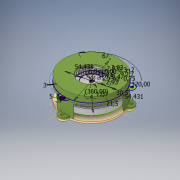
# Autodesk Inventor part: HarmonicDriveProto2
Saved by Autodesk Inventor 2018.3 (Build 223284000, 284)
## iProperties
Created: 2018-06-22
Part Number: HarmonicDriveProto2
Material: Generisch
Document SubType Name: Modeling
Designer: JochenAlt
Density: 1 g/cm^3
Appearance: Vorgabe
Author: JochenAlt
Autodesk Inventor part; units mm, degrees
note: some values were not read from the file. Chosen so that the rebuilt part matches the saved one: sketch regions of "Extrusion4".
(part 1 of 2)
ref_plane "YZ Plane" through (0, 0, 0) normal (1, 0, 0) x (0, 1, 0)
sketch "Riemen" plane through (0, 0, 0) normal (0, 0, 1) x (1, 0, 0)
  circle A0 centre (0, 0) radius 27.4555 construction
  circle A1 centre (0, 0) radius 26.4655
  circle A2 centre (0, 0) radius 29.1655 construction
  line L0 (0, 43.4877) -> (0, -41.2966) construction
  line L1 (-40.8583, 0) -> (40.8583, 0) construction
  line L2 (0, 0) -> (5.5324, 31.3756) construction
  circle A3 centre (0, 0) radius 27.2155 construction
  line L3 (-1.465, 27.176) -> (1.465, 27.176) construction
  line L4 (3.2763, 27.0176) -> (6.1618, 26.5088) construction
  arc A4 (4.2713, 28.7473) -> (3.3977, 27.4807) centre (6.1618, 26.5088) ccw
  arc A5 (0.5608, 29.1601) -> (0, 29.1655) centre (0, 0) ccw
  arc A6 (5.0645, 28.7224) -> (4.5113, 28.8145) centre (0, 0) ccw
  arc A7 (3.081, 27.2821) -> (1.7033, 27.4026) centre (0, 0) ccw
  arc A8 (1.4259, 27.6532) -> (0.7855, 29.0523) centre (-1.465, 27.176) ccw
  arc A9 (0.7855, 29.0523) -> (0.5608, 29.1601) centre (0.5551, 28.8602) ccw
  arc A10 (1.4259, 27.6532) -> (1.7033, 27.4026) centre (1.7219, 27.702) ccw
  arc A11 (3.081, 27.2821) -> (3.3977, 27.4807) centre (3.1147, 27.5802) ccw
  arc A12 (4.5113, 28.8145) -> (4.2713, 28.7473) centre (4.4649, 28.5181) ccw
  line L5 (0, 0) -> (2.7172, 31.0575) construction
  arc A13 (-4.5113, 28.8145) -> (-5.0645, 28.7224) centre (0, 0) ccw
  arc A14 (-4.2713, 28.7473) -> (-4.5113, 28.8145) centre (-4.4649, 28.5181) ccw
  arc A15 (-3.3977, 27.4807) -> (-4.2713, 28.7473) centre (-6.1618, 26.5088) ccw
  arc A16 (-1.7033, 27.4026) -> (-3.081, 27.2821) centre (0, 0) ccw
  arc A17 (-1.7033, 27.4026) -> (-1.4259, 27.6532) centre (-1.7219, 27.702) ccw
  arc A18 (-0.7855, 29.0523) -> (-1.4259, 27.6532) centre (1.465, 27.176) ccw
  arc A19 (-0.5608, 29.1601) -> (-0.7855, 29.0523) centre (-0.5551, 28.8602) ccw
  arc A20 (0, 29.1655) -> (-0.5608, 29.1601) centre (0, 0) ccw
  arc A21 (-3.3977, 27.4807) -> (-3.081, 27.2821) centre (-3.1147, 27.5802) ccw
  arc A22 (-9.4463, 27.5933) -> (-9.9752, 27.4066) centre (0, 0) ccw
  arc A23 (-9.1983, 27.5688) -> (-9.4463, 27.5933) centre (-9.3492, 27.3095) ccw
  arc A24 (-8.118, 26.4732) -> (-9.1983, 27.5688) centre (-10.6714, 25.0361) ccw
  arc A25 (-6.4358, 26.6905) -> (-7.7717, 26.3326) centre (0, 0) ccw
  arc A26 (-6.4358, 26.6905) -> (-6.2061, 26.9855) centre (-6.5061, 26.9822) ccw
  arc A27 (-5.8184, 28.4745) -> (-6.2061, 26.9855) centre (-3.2763, 27.0176) ccw
  arc A28 (-5.6159, 28.6197) -> (-5.8184, 28.4745) centre (-5.5581, 28.3253) ccw
  arc A29 (-5.0645, 28.7224) -> (-5.6159, 28.6197) centre (0, 0) ccw
  arc A30 (-8.118, 26.4732) -> (-7.7717, 26.3326) centre (-7.8566, 26.6203) ccw
  arc A31 (-14.0944, 25.5338) -> (-14.5827, 25.2581) centre (0, 0) ccw
  arc A32 (-13.8459, 25.5527) -> (-14.0944, 25.5338) centre (-13.9494, 25.2712) ccw
  arc A33 (-12.5917, 24.6613) -> (-13.8459, 25.5527) centre (-14.8567, 22.8026) ccw
  arc A34 (-10.9728, 25.1675) -> (-12.2262, 24.583) centre (0, 0) ccw
  arc A35 (-10.9728, 25.1675) -> (-10.7978, 25.4978) centre (-11.0927, 25.4425) ccw
  arc A36 (-10.6746, 27.0315) -> (-10.7978, 25.4978) centre (-7.9181, 26.0382) ccw
  arc A37 (-10.5003, 27.2097) -> (-10.6746, 27.0315) centre (-10.3923, 26.9298) ccw
  arc A38 (-9.9752, 27.4066) -> (-10.5003, 27.2097) centre (0, 0) ccw
  arc A39 (-12.5917, 24.6613) -> (-12.2262, 24.583) centre (-12.3598, 24.8516) ccw
  arc A40 (-18.3141, 22.6984) -> (-18.7472, 22.3421) centre (0, 0) ccw
  arc A41 (-18.0727, 22.7602) -> (-18.3141, 22.6984) centre (-18.1258, 22.4649) ccw
  arc A42 (-16.6828, 22.1001) -> (-18.0727, 22.7602) centre (-18.5907, 19.8764) ccw
  arc A43 (-15.1764, 22.8797) -> (-16.3093, 22.0865) centre (0, 0) ccw
  arc A44 (-15.1764, 22.8797) -> (-15.0614, 23.2354) centre (-15.3422, 23.1297) ccw
  arc A45 (-15.2064, 24.7673) -> (-15.0614, 23.2354) centre (-12.3193, 24.2676) ccw
  arc A46 (-15.0657, 24.973) -> (-15.2064, 24.7673) centre (-14.9108, 24.7161) ccw
  arc A47 (-14.5827, 25.2581) -> (-15.0657, 24.973) centre (0, 0) ccw
  arc A48 (-16.6828, 22.1001) -> (-16.3093, 22.0865) centre (-16.4875, 22.3278) ccw
  arc A49 (-21.9774, 19.1734) -> (-22.3421, 18.7472) centre (0, 0) ccw
  arc A50 (-21.7504, 19.2761) -> (-21.9774, 19.1734) centre (-21.7514, 18.9762) ccw
  arc A51 (-20.267, 18.8674) -> (-21.7504, 19.2761) centre (-21.7597, 16.3462) ccw
  arc A52 (-18.9188, 19.8968) -> (-19.8968, 18.9188) centre (0, 0) ccw
  arc A53 (-18.9188, 19.8968) -> (-18.8674, 20.267) centre (-19.1256, 20.1142) ccw
  arc A54 (-19.2761, 21.7504) -> (-18.8674, 20.267) centre (-16.3462, 21.7597) ccw
  arc A55 (-19.1734, 21.9774) -> (-19.2761, 21.7504) centre (-18.9762, 21.7514) ccw
  arc A56 (-18.7472, 22.3421) -> (-19.1734, 21.9774) centre (0, 0) ccw
  arc A57 (-20.267, 18.8674) -> (-19.8968, 18.9188) centre (-20.1142, 19.1256) ccw
  arc A58 (-24.973, 15.0657) -> (-25.2581, 14.5827) centre (0, 0) ccw
  arc A59 (-24.7673, 15.2064) -> (-24.973, 15.0657) centre (-24.7161, 14.9108) ccw
  arc A60 (-23.2354, 15.0614) -> (-24.7673, 15.2064) centre (-24.2676, 12.3193) ccw
  arc A61 (-22.0865, 16.3093) -> (-22.8797, 15.1764) centre (0, 0) ccw
  arc A62 (-22.0865, 16.3093) -> (-22.1001, 16.6828) centre (-22.3278, 16.4875) ccw
  arc A63 (-22.7602, 18.0727) -> (-22.1001, 16.6828) centre (-19.8764, 18.5907) ccw
  arc A64 (-22.6984, 18.3141) -> (-22.7602, 18.0727) centre (-22.4649, 18.1258) ccw
  arc A65 (-22.3421, 18.7472) -> (-22.6984, 18.3141) centre (0, 0) ccw
  arc A66 (-23.2354, 15.0614) -> (-22.8797, 15.1764) centre (-23.1297, 15.3422) ccw
  arc A67 (-27.2097, 10.5003) -> (-27.4066, 9.9752) centre (0, 0) ccw
  arc A68 (-27.0315, 10.6746) -> (-27.2097, 10.5003) centre (-26.9298, 10.3923) ccw
  arc A69 (-25.4978, 10.7978) -> (-27.0315, 10.6746) centre (-26.0382, 7.9181) ccw
  arc A70 (-24.583, 12.2262) -> (-25.1675, 10.9728) centre (0, 0) ccw
  arc A71 (-24.583, 12.2262) -> (-24.6613, 12.5917) centre (-24.8516, 12.3598) ccw
  arc A72 (-25.5527, 13.8459) -> (-24.6613, 12.5917) centre (-22.8026, 14.8567) ccw
  arc A73 (-25.5338, 14.0944) -> (-25.5527, 13.8459) centre (-25.2712, 13.9494) ccw
  arc A74 (-25.2581, 14.5827) -> (-25.5338, 14.0944) centre (0, 0) ccw
  arc A75 (-25.4978, 10.7978) -> (-25.1675, 10.9728) centre (-25.4425, 11.0927) ccw
  arc A76 (-28.6197, 5.6159) -> (-28.7224, 5.0645) centre (0, 0) ccw
  arc A77 (-28.4745, 5.8184) -> (-28.6197, 5.6159) centre (-28.3253, 5.5581) ccw
  arc A78 (-26.9855, 6.2061) -> (-28.4745, 5.8184) centre (-27.0176, 3.2763) ccw
  arc A79 (-26.3326, 7.7717) -> (-26.6905, 6.4358) centre (0, 0) ccw
  arc A80 (-26.3326, 7.7717) -> (-26.4732, 8.118) centre (-26.6203, 7.8566) ccw
  arc A81 (-27.5688, 9.1983) -> (-26.4732, 8.118) centre (-25.0361, 10.6714) ccw
  arc A82 (-27.5933, 9.4463) -> (-27.5688, 9.1983) centre (-27.3095, 9.3492) ccw
  arc A83 (-27.4066, 9.9752) -> (-27.5933, 9.4463) centre (0, 0) ccw
  arc A84 (-26.9855, 6.2061) -> (-26.6905, 6.4358) centre (-26.9822, 6.5061) ccw
  arc A85 (-29.1601, 0.5608) -> (-29.1655, 0) centre (0, 0) ccw
  arc A86 (-29.0523, 0.7855) -> (-29.1601, 0.5608) centre (-28.8602, 0.5551) ccw
  arc A87 (-27.6532, 1.4259) -> (-29.0523, 0.7855) centre (-27.176, -1.465) ccw
  arc A88 (-27.2821, 3.081) -> (-27.4026, 1.7033) centre (0, 0) ccw
  arc A89 (-27.2821, 3.081) -> (-27.4807, 3.3977) centre (-27.5802, 3.1147) ccw
  arc A90 (-28.7473, 4.2713) -> (-27.4807, 3.3977) centre (-26.5088, 6.1618) ccw
  arc A91 (-28.8145, 4.5113) -> (-28.7473, 4.2713) centre (-28.5181, 4.4649) ccw
  arc A92 (-28.7224, 5.0645) -> (-28.8145, 4.5113) centre (0, 0) ccw
  arc A93 (-27.6532, 1.4259) -> (-27.4026, 1.7033) centre (-27.702, 1.7219) ccw
  arc A94 (-28.8145, -4.5113) -> (-28.7224, -5.0645) centre (0, 0) ccw
  arc A95 (-28.7473, -4.2713) -> (-28.8145, -4.5113) centre (-28.5181, -4.4649) ccw
  arc A96 (-27.4807, -3.3977) -> (-28.7473, -4.2713) centre (-26.5088, -6.1618) ccw
  arc A97 (-27.4026, -1.7033) -> (-27.2821, -3.081) centre (0, 0) ccw
  arc A98 (-27.4026, -1.7033) -> (-27.6532, -1.4259) centre (-27.702, -1.7219) ccw
  arc A99 (-29.0523, -0.7855) -> (-27.6532, -1.4259) centre (-27.176, 1.465) ccw
  arc A100 (-29.1601, -0.5608) -> (-29.0523, -0.7855) centre (-28.8602, -0.5551) ccw
  arc A101 (-29.1655, 0) -> (-29.1601, -0.5608) centre (0, 0) ccw
  arc A102 (-27.4807, -3.3977) -> (-27.2821, -3.081) centre (-27.5802, -3.1147) ccw
  arc A103 (-27.5933, -9.4463) -> (-27.4066, -9.9752) centre (0, 0) ccw
  arc A104 (-27.5688, -9.1983) -> (-27.5933, -9.4463) centre (-27.3095, -9.3492) ccw
  arc A105 (-26.4732, -8.118) -> (-27.5688, -9.1983) centre (-25.0361, -10.6714) ccw
  arc A106 (-26.6905, -6.4358) -> (-26.3326, -7.7717) centre (0, 0) ccw
  arc A107 (-26.6905, -6.4358) -> (-26.9855, -6.2061) centre (-26.9822, -6.5061) ccw
  arc A108 (-28.4745, -5.8184) -> (-26.9855, -6.2061) centre (-27.0176, -3.2763) ccw
  arc A109 (-28.6197, -5.6159) -> (-28.4745, -5.8184) centre (-28.3253, -5.5581) ccw
  arc A110 (-28.7224, -5.0645) -> (-28.6197, -5.6159) centre (0, 0) ccw
  arc A111 (-26.4732, -8.118) -> (-26.3326, -7.7717) centre (-26.6203, -7.8566) ccw
  arc A112 (-25.5338, -14.0944) -> (-25.2581, -14.5827) centre (0, 0) ccw
  arc A113 (-25.5527, -13.8459) -> (-25.5338, -14.0944) centre (-25.2712, -13.9494) ccw
  arc A114 (-24.6613, -12.5917) -> (-25.5527, -13.8459) centre (-22.8026, -14.8567) ccw
  arc A115 (-25.1675, -10.9728) -> (-24.583, -12.2262) centre (0, 0) ccw
  arc A116 (-25.1675, -10.9728) -> (-25.4978, -10.7978) centre (-25.4425, -11.0927) ccw
  arc A117 (-27.0315, -10.6746) -> (-25.4978, -10.7978) centre (-26.0382, -7.9181) ccw
  arc A118 (-27.2097, -10.5003) -> (-27.0315, -10.6746) centre (-26.9298, -10.3923) ccw
  arc A119 (-27.4066, -9.9752) -> (-27.2097, -10.5003) centre (0, 0) ccw
  arc A120 (-24.6613, -12.5917) -> (-24.583, -12.2262) centre (-24.8516, -12.3598) ccw
  arc A121 (-22.6984, -18.3141) -> (-22.3421, -18.7472) centre (0, 0) ccw
  arc A122 (-22.7602, -18.0727) -> (-22.6984, -18.3141) centre (-22.4649, -18.1258) ccw
  arc A123 (-22.1001, -16.6828) -> (-22.7602, -18.0727) centre (-19.8764, -18.5907) ccw
  arc A124 (-22.8797, -15.1764) -> (-22.0865, -16.3093) centre (0, 0) ccw
  arc A125 (-22.8797, -15.1764) -> (-23.2354, -15.0614) centre (-23.1297, -15.3422) ccw
  arc A126 (-24.7673, -15.2064) -> (-23.2354, -15.0614) centre (-24.2676, -12.3193) ccw
  arc A127 (-24.973, -15.0657) -> (-24.7673, -15.2064) centre (-24.7161, -14.9108) ccw
  arc A128 (-25.2581, -14.5827) -> (-24.973, -15.0657) centre (0, 0) ccw
  arc A129 (-22.1001, -16.6828) -> (-22.0865, -16.3093) centre (-22.3278, -16.4875) ccw
  arc A130 (-19.1734, -21.9774) -> (-18.7472, -22.3421) centre (0, 0) ccw
  arc A131 (-19.2761, -21.7504) -> (-19.1734, -21.9774) centre (-18.9762, -21.7514) ccw
  arc A132 (-18.8674, -20.267) -> (-19.2761, -21.7504) centre (-16.3462, -21.7597) ccw
  arc A133 (-19.8968, -18.9188) -> (-18.9188, -19.8968) centre (0, 0) ccw
  arc A134 (-19.8968, -18.9188) -> (-20.267, -18.8674) centre (-20.1142, -19.1256) ccw
  arc A135 (-21.7504, -19.2761) -> (-20.267, -18.8674) centre (-21.7597, -16.3462) ccw
  arc A136 (-21.9774, -19.1734) -> (-21.7504, -19.2761) centre (-21.7514, -18.9762) ccw
  arc A137 (-22.3421, -18.7472) -> (-21.9774, -19.1734) centre (0, 0) ccw
  arc A138 (-18.8674, -20.267) -> (-18.9188, -19.8968) centre (-19.1256, -20.1142) ccw
  arc A139 (-15.0657, -24.973) -> (-14.5827, -25.2581) centre (0, 0) ccw
  arc A140 (-15.2064, -24.7673) -> (-15.0657, -24.973) centre (-14.9108, -24.7161) ccw
  arc A141 (-15.0614, -23.2354) -> (-15.2064, -24.7673) centre (-12.3193, -24.2676) ccw
  arc A142 (-16.3093, -22.0865) -> (-15.1764, -22.8797) centre (0, 0) ccw
  arc A143 (-16.3093, -22.0865) -> (-16.6828, -22.1001) centre (-16.4875, -22.3278) ccw
  arc A144 (-18.0727, -22.7602) -> (-16.6828, -22.1001) centre (-18.5907, -19.8764) ccw
  arc A145 (-18.3141, -22.6984) -> (-18.0727, -22.7602) centre (-18.1258, -22.4649) ccw
  arc A146 (-18.7472, -22.3421) -> (-18.3141, -22.6984) centre (0, 0) ccw
  arc A147 (-15.0614, -23.2354) -> (-15.1764, -22.8797) centre (-15.3422, -23.1297) ccw
  arc A148 (-10.5003, -27.2097) -> (-9.9752, -27.4066) centre (0, 0) ccw
  arc A149 (-10.6746, -27.0315) -> (-10.5003, -27.2097) centre (-10.3923, -26.9298) ccw
  arc A150 (-10.7978, -25.4978) -> (-10.6746, -27.0315) centre (-7.9181, -26.0382) ccw
  arc A151 (-12.2262, -24.583) -> (-10.9728, -25.1675) centre (0, 0) ccw
  arc A152 (-12.2262, -24.583) -> (-12.5917, -24.6613) centre (-12.3598, -24.8516) ccw
  arc A153 (-13.8459, -25.5527) -> (-12.5917, -24.6613) centre (-14.8567, -22.8026) ccw
  arc A154 (-14.0944, -25.5338) -> (-13.8459, -25.5527) centre (-13.9494, -25.2712) ccw
  arc A155 (-14.5827, -25.2581) -> (-14.0944, -25.5338) centre (0, 0) ccw
  arc A156 (-10.7978, -25.4978) -> (-10.9728, -25.1675) centre (-11.0927, -25.4425) ccw
  arc A157 (-5.6159, -28.6197) -> (-5.0645, -28.7224) centre (0, 0) ccw
  arc A158 (-5.8184, -28.4745) -> (-5.6159, -28.6197) centre (-5.5581, -28.3253) ccw
  arc A159 (-6.2061, -26.9855) -> (-5.8184, -28.4745) centre (-3.2763, -27.0176) ccw
  arc A160 (-7.7717, -26.3326) -> (-6.4358, -26.6905) centre (0, 0) ccw
  arc A161 (-7.7717, -26.3326) -> (-8.118, -26.4732) centre (-7.8566, -26.6203) ccw
  arc A162 (-9.1983, -27.5688) -> (-8.118, -26.4732) centre (-10.6714, -25.0361) ccw
  arc A163 (-9.4463, -27.5933) -> (-9.1983, -27.5688) centre (-9.3492, -27.3095) ccw
  arc A164 (-9.9752, -27.4066) -> (-9.4463, -27.5933) centre (0, 0) ccw
  arc A165 (-6.2061, -26.9855) -> (-6.4358, -26.6905) centre (-6.5061, -26.9822) ccw
  arc A166 (-0.5608, -29.1601) -> (0, -29.1655) centre (0, 0) ccw
  arc A167 (-0.7855, -29.0523) -> (-0.5608, -29.1601) centre (-0.5551, -28.8602) ccw
  arc A168 (-1.4259, -27.6532) -> (-0.7855, -29.0523) centre (1.465, -27.176) ccw
  arc A169 (-3.081, -27.2821) -> (-1.7033, -27.4026) centre (0, 0) ccw
  arc A170 (-3.081, -27.2821) -> (-3.3977, -27.4807) centre (-3.1147, -27.5802) ccw
  arc A171 (-4.2713, -28.7473) -> (-3.3977, -27.4807) centre (-6.1618, -26.5088) ccw
  arc A172 (-4.5113, -28.8145) -> (-4.2713, -28.7473) centre (-4.4649, -28.5181) ccw
  arc A173 (-5.0645, -28.7224) -> (-4.5113, -28.8145) centre (0, 0) ccw
  arc A174 (-1.4259, -27.6532) -> (-1.7033, -27.4026) centre (-1.7219, -27.702) ccw
  arc A175 (4.5113, -28.8145) -> (5.0645, -28.7224) centre (0, 0) ccw
  arc A176 (4.2713, -28.7473) -> (4.5113, -28.8145) centre (4.4649, -28.5181) ccw
  arc A177 (3.3977, -27.4807) -> (4.2713, -28.7473) centre (6.1618, -26.5088) ccw
  arc A178 (1.7033, -27.4026) -> (3.081, -27.2821) centre (0, 0) ccw
  arc A179 (1.7033, -27.4026) -> (1.4259, -27.6532) centre (1.7219, -27.702) ccw
  arc A180 (0.7855, -29.0523) -> (1.4259, -27.6532) centre (-1.465, -27.176) ccw
  arc A181 (0.5608, -29.1601) -> (0.7855, -29.0523) centre (0.5551, -28.8602) ccw
  arc A182 (0, -29.1655) -> (0.5608, -29.1601) centre (0, 0) ccw
  arc A183 (3.3977, -27.4807) -> (3.081, -27.2821) centre (3.1147, -27.5802) ccw
  arc A184 (9.4463, -27.5933) -> (9.9752, -27.4066) centre (0, 0) ccw
  arc A185 (9.1983, -27.5688) -> (9.4463, -27.5933) centre (9.3492, -27.3095) ccw
  arc A186 (8.118, -26.4732) -> (9.1983, -27.5688) centre (10.6714, -25.0361) ccw
  arc A187 (6.4358, -26.6905) -> (7.7717, -26.3326) centre (0, 0) ccw
  arc A188 (6.4358, -26.6905) -> (6.2061, -26.9855) centre (6.5061, -26.9822) ccw
  arc A189 (5.8184, -28.4745) -> (6.2061, -26.9855) centre (3.2763, -27.0176) ccw
  arc A190 (5.6159, -28.6197) -> (5.8184, -28.4745) centre (5.5581, -28.3253) ccw
  arc A191 (5.0645, -28.7224) -> (5.6159, -28.6197) centre (0, 0) ccw
  arc A192 (8.118, -26.4732) -> (7.7717, -26.3326) centre (7.8566, -26.6203) ccw
  arc A193 (14.0944, -25.5338) -> (14.5827, -25.2581) centre (0, 0) ccw
  arc A194 (13.8459, -25.5527) -> (14.0944, -25.5338) centre (13.9494, -25.2712) ccw
  arc A195 (12.5917, -24.6613) -> (13.8459, -25.5527) centre (14.8567, -22.8026) ccw
  arc A196 (10.9728, -25.1675) -> (12.2262, -24.583) centre (0, 0) ccw
  arc A197 (10.9728, -25.1675) -> (10.7978, -25.4978) centre (11.0927, -25.4425) ccw
  arc A198 (10.6746, -27.0315) -> (10.7978, -25.4978) centre (7.9181, -26.0382) ccw
  arc A199 (10.5003, -27.2097) -> (10.6746, -27.0315) centre (10.3923, -26.9298) ccw
  arc A200 (9.9752, -27.4066) -> (10.5003, -27.2097) centre (0, 0) ccw
  arc A201 (12.5917, -24.6613) -> (12.2262, -24.583) centre (12.3598, -24.8516) ccw
  arc A202 (18.3141, -22.6984) -> (18.7472, -22.3421) centre (0, 0) ccw
  arc A203 (18.0727, -22.7602) -> (18.3141, -22.6984) centre (18.1258, -22.4649) ccw
  arc A204 (16.6828, -22.1001) -> (18.0727, -22.7602) centre (18.5907, -19.8764) ccw
  arc A205 (15.1764, -22.8797) -> (16.3093, -22.0865) centre (0, 0) ccw
  arc A206 (15.1764, -22.8797) -> (15.0614, -23.2354) centre (15.3422, -23.1297) ccw
  arc A207 (15.2064, -24.7673) -> (15.0614, -23.2354) centre (12.3193, -24.2676) ccw
  arc A208 (15.0657, -24.973) -> (15.2064, -24.7673) centre (14.9108, -24.7161) ccw
  arc A209 (14.5827, -25.2581) -> (15.0657, -24.973) centre (0, 0) ccw
  arc A210 (16.6828, -22.1001) -> (16.3093, -22.0865) centre (16.4875, -22.3278) ccw
  arc A211 (21.9774, -19.1734) -> (22.3421, -18.7472) centre (0, 0) ccw
  arc A212 (21.7504, -19.2761) -> (21.9774, -19.1734) centre (21.7514, -18.9762) ccw
  arc A213 (20.267, -18.8674) -> (21.7504, -19.2761) centre (21.7597, -16.3462) ccw
  arc A214 (18.9188, -19.8968) -> (19.8968, -18.9188) centre (0, 0) ccw
  arc A215 (18.9188, -19.8968) -> (18.8674, -20.267) centre (19.1256, -20.1142) ccw
  arc A216 (19.2761, -21.7504) -> (18.8674, -20.267) centre (16.3462, -21.7597) ccw
  arc A217 (19.1734, -21.9774) -> (19.2761, -21.7504) centre (18.9762, -21.7514) ccw
  arc A218 (18.7472, -22.3421) -> (19.1734, -21.9774) centre (0, 0) ccw
  arc A219 (20.267, -18.8674) -> (19.8968, -18.9188) centre (20.1142, -19.1256) ccw
  arc A220 (24.973, -15.0657) -> (25.2581, -14.5827) centre (0, 0) ccw
  arc A221 (24.7673, -15.2064) -> (24.973, -15.0657) centre (24.7161, -14.9108) ccw
  arc A222 (23.2354, -15.0614) -> (24.7673, -15.2064) centre (24.2676, -12.3193) ccw
  arc A223 (22.0865, -16.3093) -> (22.8797, -15.1764) centre (0, 0) ccw
  arc A224 (22.0865, -16.3093) -> (22.1001, -16.6828) centre (22.3278, -16.4875) ccw
  arc A225 (22.7602, -18.0727) -> (22.1001, -16.6828) centre (19.8764, -18.5907) ccw
  arc A226 (22.6984, -18.3141) -> (22.7602, -18.0727) centre (22.4649, -18.1258) ccw
  arc A227 (22.3421, -18.7472) -> (22.6984, -18.3141) centre (0, 0) ccw
  arc A228 (23.2354, -15.0614) -> (22.8797, -15.1764) centre (23.1297, -15.3422) ccw
  arc A229 (27.2097, -10.5003) -> (27.4066, -9.9752) centre (0, 0) ccw
  arc A230 (27.0315, -10.6746) -> (27.2097, -10.5003) centre (26.9298, -10.3923) ccw
  arc A231 (25.4978, -10.7978) -> (27.0315, -10.6746) centre (26.0382, -7.9181) ccw
  arc A232 (24.583, -12.2262) -> (25.1675, -10.9728) centre (0, 0) ccw
  arc A233 (24.583, -12.2262) -> (24.6613, -12.5917) centre (24.8516, -12.3598) ccw
  arc A234 (25.5527, -13.8459) -> (24.6613, -12.5917) centre (22.8026, -14.8567) ccw
  arc A235 (25.5338, -14.0944) -> (25.5527, -13.8459) centre (25.2712, -13.9494) ccw
  arc A236 (25.2581, -14.5827) -> (25.5338, -14.0944) centre (0, 0) ccw
  arc A237 (25.4978, -10.7978) -> (25.1675, -10.9728) centre (25.4425, -11.0927) ccw
  arc A238 (28.6197, -5.6159) -> (28.7224, -5.0645) centre (0, 0) ccw
  arc A239 (28.4745, -5.8184) -> (28.6197, -5.6159) centre (28.3253, -5.5581) ccw
  arc A240 (26.9855, -6.2061) -> (28.4745, -5.8184) centre (27.0176, -3.2763) ccw
  arc A241 (26.3326, -7.7717) -> (26.6905, -6.4358) centre (0, 0) ccw
  arc A242 (26.3326, -7.7717) -> (26.4732, -8.118) centre (26.6203, -7.8566) ccw
  arc A243 (27.5688, -9.1983) -> (26.4732, -8.118) centre (25.0361, -10.6714) ccw
  arc A244 (27.5933, -9.4463) -> (27.5688, -9.1983) centre (27.3095, -9.3492) ccw
  arc A245 (27.4066, -9.9752) -> (27.5933, -9.4463) centre (0, 0) ccw
  arc A246 (26.9855, -6.2061) -> (26.6905, -6.4358) centre (26.9822, -6.5061) ccw
  arc A247 (29.1601, -0.5608) -> (29.1655, 0) centre (0, 0) ccw
  arc A248 (29.0523, -0.7855) -> (29.1601, -0.5608) centre (28.8602, -0.5551) ccw
  arc A249 (27.6532, -1.4259) -> (29.0523, -0.7855) centre (27.176, 1.465) ccw
  arc A250 (27.2821, -3.081) -> (27.4026, -1.7033) centre (0, 0) ccw
  arc A251 (27.2821, -3.081) -> (27.4807, -3.3977) centre (27.5802, -3.1147) ccw
  arc A252 (28.7473, -4.2713) -> (27.4807, -3.3977) centre (26.5088, -6.1618) ccw
  arc A253 (28.8145, -4.5113) -> (28.7473, -4.2713) centre (28.5181, -4.4649) ccw
  arc A254 (28.7224, -5.0645) -> (28.8145, -4.5113) centre (0, 0) ccw
  arc A255 (27.6532, -1.4259) -> (27.4026, -1.7033) centre (27.702, -1.7219) ccw
  arc A256 (28.8145, 4.5113) -> (28.7224, 5.0645) centre (0, 0) ccw
  arc A257 (28.7473, 4.2713) -> (28.8145, 4.5113) centre (28.5181, 4.4649) ccw
  arc A258 (27.4807, 3.3977) -> (28.7473, 4.2713) centre (26.5088, 6.1618) ccw
  arc A259 (27.4026, 1.7033) -> (27.2821, 3.081) centre (0, 0) ccw
  arc A260 (27.4026, 1.7033) -> (27.6532, 1.4259) centre (27.702, 1.7219) ccw
  arc A261 (29.0523, 0.7855) -> (27.6532, 1.4259) centre (27.176, -1.465) ccw
  arc A262 (29.1601, 0.5608) -> (29.0523, 0.7855) centre (28.8602, 0.5551) ccw
  arc A263 (29.1655, 0) -> (29.1601, 0.5608) centre (0, 0) ccw
  arc A264 (27.4807, 3.3977) -> (27.2821, 3.081) centre (27.5802, 3.1147) ccw
  arc A265 (27.5933, 9.4463) -> (27.4066, 9.9752) centre (0, 0) ccw
  arc A266 (27.5688, 9.1983) -> (27.5933, 9.4463) centre (27.3095, 9.3492) ccw
  arc A267 (26.4732, 8.118) -> (27.5688, 9.1983) centre (25.0361, 10.6714) ccw
  arc A268 (26.6905, 6.4358) -> (26.3326, 7.7717) centre (0, 0) ccw
  arc A269 (26.6905, 6.4358) -> (26.9855, 6.2061) centre (26.9822, 6.5061) ccw
  arc A270 (28.4745, 5.8184) -> (26.9855, 6.2061) centre (27.0176, 3.2763) ccw
  arc A271 (28.6197, 5.6159) -> (28.4745, 5.8184) centre (28.3253, 5.5581) ccw
  arc A272 (28.7224, 5.0645) -> (28.6197, 5.6159) centre (0, 0) ccw
  arc A273 (26.4732, 8.118) -> (26.3326, 7.7717) centre (26.6203, 7.8566) ccw
  arc A274 (25.5338, 14.0944) -> (25.2581, 14.5827) centre (0, 0) ccw
  arc A275 (25.5527, 13.8459) -> (25.5338, 14.0944) centre (25.2712, 13.9494) ccw
  arc A276 (24.6613, 12.5917) -> (25.5527, 13.8459) centre (22.8026, 14.8567) ccw
  arc A277 (25.1675, 10.9728) -> (24.583, 12.2262) centre (0, 0) ccw
  arc A278 (25.1675, 10.9728) -> (25.4978, 10.7978) centre (25.4425, 11.0927) ccw
  arc A279 (27.0315, 10.6746) -> (25.4978, 10.7978) centre (26.0382, 7.9181) ccw
  arc A280 (27.2097, 10.5003) -> (27.0315, 10.6746) centre (26.9298, 10.3923) ccw
  arc A281 (27.4066, 9.9752) -> (27.2097, 10.5003) centre (0, 0) ccw
  arc A282 (24.6613, 12.5917) -> (24.583, 12.2262) centre (24.8516, 12.3598) ccw
  arc A283 (22.6984, 18.3141) -> (22.3421, 18.7472) centre (0, 0) ccw
  arc A284 (22.7602, 18.0727) -> (22.6984, 18.3141) centre (22.4649, 18.1258) ccw
  arc A285 (22.1001, 16.6828) -> (22.7602, 18.0727) centre (19.8764, 18.5907) ccw
  arc A286 (22.8797, 15.1764) -> (22.0865, 16.3093) centre (0, 0) ccw
  arc A287 (22.8797, 15.1764) -> (23.2354, 15.0614) centre (23.1297, 15.3422) ccw
  arc A288 (24.7673, 15.2064) -> (23.2354, 15.0614) centre (24.2676, 12.3193) ccw
  arc A289 (24.973, 15.0657) -> (24.7673, 15.2064) centre (24.7161, 14.9108) ccw
  arc A290 (25.2581, 14.5827) -> (24.973, 15.0657) centre (0, 0) ccw
  arc A291 (22.1001, 16.6828) -> (22.0865, 16.3093) centre (22.3278, 16.4875) ccw
  arc A292 (19.1734, 21.9774) -> (18.7472, 22.3421) centre (0, 0) ccw
  arc A293 (19.2761, 21.7504) -> (19.1734, 21.9774) centre (18.9762, 21.7514) ccw
  arc A294 (18.8674, 20.267) -> (19.2761, 21.7504) centre (16.3462, 21.7597) ccw
  arc A295 (19.8968, 18.9188) -> (18.9188, 19.8968) centre (0, 0) ccw
  arc A296 (19.8968, 18.9188) -> (20.267, 18.8674) centre (20.1142, 19.1256) ccw
  arc A297 (21.7504, 19.2761) -> (20.267, 18.8674) centre (21.7597, 16.3462) ccw
  arc A298 (21.9774, 19.1734) -> (21.7504, 19.2761) centre (21.7514, 18.9762) ccw
  arc A299 (22.3421, 18.7472) -> (21.9774, 19.1734) centre (0, 0) ccw
  arc A300 (18.8674, 20.267) -> (18.9188, 19.8968) centre (19.1256, 20.1142) ccw
  arc A301 (15.0657, 24.973) -> (14.5827, 25.2581) centre (0, 0) ccw
  arc A302 (15.2064, 24.7673) -> (15.0657, 24.973) centre (14.9108, 24.7161) ccw
  arc A303 (15.0614, 23.2354) -> (15.2064, 24.7673) centre (12.3193, 24.2676) ccw
  arc A304 (16.3093, 22.0865) -> (15.1764, 22.8797) centre (0, 0) ccw
  arc A305 (16.3093, 22.0865) -> (16.6828, 22.1001) centre (16.4875, 22.3278) ccw
  arc A306 (18.0727, 22.7602) -> (16.6828, 22.1001) centre (18.5907, 19.8764) ccw
  arc A307 (18.3141, 22.6984) -> (18.0727, 22.7602) centre (18.1258, 22.4649) ccw
  arc A308 (18.7472, 22.3421) -> (18.3141, 22.6984) centre (0, 0) ccw
  arc A309 (15.0614, 23.2354) -> (15.1764, 22.8797) centre (15.3422, 23.1297) ccw
  arc A310 (10.5003, 27.2097) -> (9.9752, 27.4066) centre (0, 0) ccw
  arc A311 (10.6746, 27.0315) -> (10.5003, 27.2097) centre (10.3923, 26.9298) ccw
  arc A312 (10.7978, 25.4978) -> (10.6746, 27.0315) centre (7.9181, 26.0382) ccw
  arc A313 (12.2262, 24.583) -> (10.9728, 25.1675) centre (0, 0) ccw
  arc A314 (12.2262, 24.583) -> (12.5917, 24.6613) centre (12.3598, 24.8516) ccw
  arc A315 (13.8459, 25.5527) -> (12.5917, 24.6613) centre (14.8567, 22.8026) ccw
  arc A316 (14.0944, 25.5338) -> (13.8459, 25.5527) centre (13.9494, 25.2712) ccw
  arc A317 (14.5827, 25.2581) -> (14.0944, 25.5338) centre (0, 0) ccw
  arc A318 (10.7978, 25.4978) -> (10.9728, 25.1675) centre (11.0927, 25.4425) ccw
  arc A319 (5.6159, 28.6197) -> (5.0645, 28.7224) centre (0, 0) ccw
  arc A320 (5.8184, 28.4745) -> (5.6159, 28.6197) centre (5.5581, 28.3253) ccw
  arc A321 (6.2061, 26.9855) -> (5.8184, 28.4745) centre (3.2763, 27.0176) ccw
  arc A322 (7.7717, 26.3326) -> (6.4358, 26.6905) centre (0, 0) ccw
  arc A323 (7.7717, 26.3326) -> (8.118, 26.4732) centre (7.8566, 26.6203) ccw
  arc A324 (9.1983, 27.5688) -> (8.118, 26.4732) centre (10.6714, 25.0361) ccw
  arc A325 (9.4463, 27.5933) -> (9.1983, 27.5688) centre (9.3492, 27.3095) ccw
  arc A326 (9.9752, 27.4066) -> (9.4463, 27.5933) centre (0, 0) ccw
  arc A327 (6.2061, 26.9855) -> (6.4358, 26.6905) centre (6.5061, 26.9822) ccw
  point P0 (0, 27.4555)
  point P1 (4.7676, 27.0384)
  dimension "d0" = 10
  dimension "d258" = 1.71
  dimension "d259" = 2.7
  dimension "d260" = 0.75
  dimension "d261" = 54.431
  dimension "d262" = 2.93
  dimension "d264" = 0.3
  dimension "d265" = 2.93
  constraints: 660 point on circle, 328 centre point, 8 end point, 8 tangent, 6 coincident, 6 equal radius, 4 point on line, 1 equal length, 1 horizontal, 1 symmetric about line, 2 other
  measures "d0" angle of L2 L0
  measures "d258" radial gap between concentric circles of A2 A0
  measures "d259" radial gap between concentric circles of A2 A1
  measures "d260" radial gap between concentric circles of A3 A1
  measures "d261" diameter of A3
  measures "d262" distance of L3.start L3.end
  measures "d264" radius of A9
  measures "d265" radius of A8
sketch "Enclosure" plane through (0, 0, 0) normal (0, 0, 1) x (1, 0, 0)
  circle A0 centre (0, 0) radius 2
  circle A1 centre (0, 0) radius 33.5
  circle A2 centre (0, 0) radius 15.25
  circle A3 centre (0, 0) radius 31.5
  line L0 (0, 51.8) -> (0, -55.3) construction
  circle A4 centre (0, -36.5) radius 1.5
  circle A5 centre (-31.6099, 18.25) radius 1.5
  circle A6 centre (31.6099, 18.25) radius 1.5
  circle A7 centre (0, 0) radius 36.5 construction
  line L1 (5.5282, -31.0111) -> (5.8792, -32.9801) construction
  line L2 (-5.5282, -31.0111) -> (-5.8792, -32.9801) construction
  circle A8 centre (31.6099, 18.25) radius 2.5
  circle A9 centre (-31.6099, 18.25) radius 2.5
  circle A10 centre (0, -36.5) radius 2.5
  line L3 (0, 0) -> (-31.6099, 18.25) construction
  line L4 (31.6099, 18.25) -> (0, 0) construction
  arc A11 (-5.8792, -32.9801) -> (5.8792, -32.9801) centre (0, -34.0281) ccw
  line L5 (0, -39) -> (0, -40) construction
  arc A12 (-25.622, 21.5816) -> (-31.5012, 11.3985) centre (-29.4692, 17.0141) ccw
  line L6 (-25.622, 21.5816) -> (-24.0923, 20.2931) construction
  line L7 (-31.5012, 11.3985) -> (-29.6205, 10.718) construction
  arc A13 (31.5012, 11.3985) -> (25.622, 21.5816) centre (29.4692, 17.0141) ccw
  circle A14 centre (0, 0) radius 34.0281 construction
  circle A15 centre (0, 0) radius 10.75
  dimension "d101" = 5
  dimension "d12" = 67
  dimension "d13" = 4
  dimension "d14" = 30.5
  dimension "d19" = 2
  dimension "d35" = 3
  dimension "d36" = 3
  dimension "d181" = 1
  dimension "d182" = 120
  dimension "d191" = 21.5
  constraints: 22 point on circle, 15 centre point, 14 end point, 10 coincident, 6 point on line, 5 equal radius, 4 tangent, 1 vertical alignment, 4 other
  measures "d12" diameter of A1
  measures "d13" diameter of A0
  measures "d14" diameter of A2
  measures "d19" radial gap between concentric circles of A1 A3
  measures "d35" diameter of A4
  measures "d36" radial gap between concentric circles of A7 A1
  measures "d181" distance of L5.end L5.start
  measures "d182" angle of L4 L3
  measures "d191" diameter of A15
extrude "Extrusion1" add sketch "Enclosure" along normal blind 7 contours A1 | A3
extrude "Extrusion2" cut sketch "Riemen" along normal blind 5 contours A1 | A12 A6 A319 A320 A321 A327 A322 A323 A324 A325 A326 A310 A311 A312 A318 A313 A314 A315 A316 A317 A301 A302 A303 A309 A304 A305 A306 A307 A308 A292 A293 A294 A300 A295 A296 A297 A298 A299 A283 A284 A285 A291 A286 A287 A288 A289 A290 A274 A275 A276 A282 A277 A278 A279 A280 A281 A265 A266 A267 A273 A268 A269 A270 A271 A272 A256 A257 A258 A264 A259 A260 A261 A262 A263 A247 A248 A249 A255 A250 A251 A252 A253 A254 A238 A239 A240 A246 A241 A242 A243 A244 A245 A229 A230 A231 A237 A232 A233 A234 A235 A236 A220 A221 A222 A228 A223 A224 A225 A226 A227 A211 A212 A213 A219 A214 A215 A216 A217 A218 A202 A203 A204 A210 A205 A206 A207 A208 A209 A193 A194 A195 A201 A196 A197 A198 A199 A200 A184 A185 A186 A192 A187 A188 A189 A190 A191 A175 A176 A177 A183 A178 A179 A180 A181 A182 A166 A167 A168 A174 A169 A170 A171 A172 A173 A157 A158 A159 A165 A160 A161 A162 A163 A164 A148 A149 A150 A156 A151 A152 A153 A154 A155 A139 A140 A141 A147 A142 A143 A144 A145 A146 A130 A131 A132 A138 A133 A134 A135 A136 A137 A121 A122 A123 A129 A124 A125 A126 A127 A128 A112 A113 A114 A120 A115 A116 A117 A118 A119 A103 A104 A105 A111 A106 A107 A108 A109 A110 A94 A95 A96 A102 A97 A98 A99 A100 A101 A85 A86 A87 A93 A88 A89 A90 A91 A92 A76 A77 A78 A84 A79 A80 A81 A82 A83 A67 A68 A69 A75 A70 A71 A72 A73 A74 A58 A59 A60 A66 A61 A62 A63 A64 A65 A49 A50 A51 A57 A52 A53 A54 A55 A56 A40 A41 A42 A48 A43 A44 A45 A46 A47 A31 A32 A33 A39 A34 A35 A36 A37 A38 A22 A23 A24 A30 A25 A26 A27 A28 A29 A13 A14 A15 A21 A16 A17 A18 A19 A20 A5 A9 A8 A10 A7 A11 A4
ref_plane "Arbeitsebene1" through (0, 0, -20) normal (0, 0, 1) x (1, 0, 0)
extrude "Extrusion7" add sketch "Enclosure" along normal blind 2 from surface at -20 contours A1 A13 | A11 A1 | A1 A12 | A8 | A9 | A10
sketch "Skizze4" plane through (0, 0, -20) normal (0, 0, -1) x (-1, 0, 0)
  circle A0 centre (0, 0) radius 10.5
  circle A1 centre (0, 0) radius 9.5
  circle A2 centre (0, 0) radius 5
  circle A3 centre (0, 0) radius 33.5 projected
  circle A4 centre (0, 0) radius 33.5 projected
  circle A5 centre (0, 0) radius 33.5 projected
  circle A6 centre (0, 0) radius 33.5 projected
  circle A7 centre (0, 0) radius 33.5 projected
  arc A8 (-33.5, 0) -> (-33.5, 0) centre (-32.1073, 5.7113) ccw
  circle A9 centre (-31.6099, 18.25) radius 1.5 projected
  circle A10 centre (0, -36.5) radius 1.5 projected
  circle A11 centre (31.6099, 18.25) radius 1.5 projected
  line L0 (0, -54.7) -> (0, 48.2) construction
  line L1 (-52.6777, 0) -> (52.6777, 0) construction
  arc A12 (-33.5, 0) -> (-33.5, 0) centre (-32.1073, 5.7113) ccw
  arc A13 (31.5012, 11.3985) -> (25.622, 21.5816) centre (29.4692, 17.0141) ccw projected
  arc A14 (-25.622, 21.5816) -> (-31.5012, 11.3985) centre (-29.4692, 17.0141) ccw projected
  arc A15 (-5.8792, -32.9801) -> (5.8792, -32.9801) centre (0, -34.0281) ccw projected
  circle A16 centre (0, -36.5) radius 2.5 projected
  circle A17 centre (-31.6099, 18.25) radius 2.5 projected
  circle A18 centre (31.6099, 18.25) radius 2.5 projected
  circle A19 centre (0, 0) radius 33.5 projected
  circle A20 centre (0, 0) radius 31.5 projected
  line L2 (29.2902, -18.23) -> (28.4413, -17.7016) construction
  point P0 (0, 33.5)
  dimension "d22" = 21
  dimension "d23" = 19
  dimension "d45" = 10
  dimension "d241" = 1
  constraints: 5 centre point, 4 point on circle, 3 coincident, 2 end point, 1 point on line, 4 other
  measures "d22" diameter of A0
  measures "d23" diameter of A1
  measures "d45" diameter of A2
  measures "d241" distance of L2.start L2.end
extrude "Extrusion4" add sketch "Skizze4" along normal blind 2 separate body contours A3 A8 A20 | A3 A13 | A15 A3 | A3 A8 A14 | A3 A8 A20 | A3 A14 A8 | A20 A8 | A8 A20 | A16 | A17 | A18 picked at (-28.0603, 20.0861) picked at (-31.5858, 11.4923)
extrude "Extrusion5" add sketch "Skizze4" along normal blind 5 contours A0 bodies 2
extrude "Extrusion6" add sketch "Skizze4" against normal blind 4 from surface at 5 contours A0 | A1 bodies 2
extrude "Extrusion8" add sketch "Enclosure" against normal up to surface (20 mm away) contours A1 bodies 1
ref_plane "Arbeitsebene10" through (0, 0, -16) normal (0, 0, 1) x (1, 0, 0)
sketch "Holes" plane through (0, 0, -16) normal (0, 0, 1) x (1, 0, 0)
  line L0 (0, 250.5339) -> (0, -318.2557) construction
  line L1 (-57.6228, 0) -> (60.6692, 0) construction
  line L2 (-22.5, 35.1536) -> (22.5, 35.1536)
  line L3 (-19.1939, -37.0624) -> (-41.6939, 1.9088)
  line L4 (41.6939, 1.9088) -> (19.1939, -37.0624)
  line L5 (-22.5, 12.9904) -> (-22.5, 35.1536)
  line L6 (22.5, 35.1536) -> (22.5, 12.9904)
  circle A0 centre (0, 0) radius 33.5 construction
  line L7 (-41.6939, 1.9088) -> (-22.5, 12.9904)
  line L8 (-19.1939, -37.0624) -> (0, -25.9808)
  line L9 (19.1939, -37.0624) -> (0, -25.9808)
  line L10 (41.6939, 1.9088) -> (22.5, 12.9904)
  line L11 (0, -25.9808) -> (22.5, 12.9904) construction
  line L12 (0, -25.9808) -> (-22.5, 12.9904) construction
  line L13 (0, 0) -> (22.5, 12.9904) construction
  line L14 (-11.25, -6.4952) -> (0, 0) construction
  circle A1 centre (0, 0) radius 25.9808
  dimension "d123" = 45
  constraints: 26 end point, 6 perpendicular, 4 equal length, 3 point on circle, 1 centre point, 1 coincident, 1 collinear, 1 midpoint, 1 parallel, 1 point on line, 1 other
  measures "d123" distance of L2.start L2.end
extrude "Extrusion33" cut sketch "Holes" along normal mid plane 25 contours L2 L6 A1 L5 | A1 L8 L3 L7 | L10 L4 L9 A1 bodies 1
ref_plane "Arbeitsebene13" through (0, 0, -15) normal (0, 0, -1) x (-1, 0, 0)